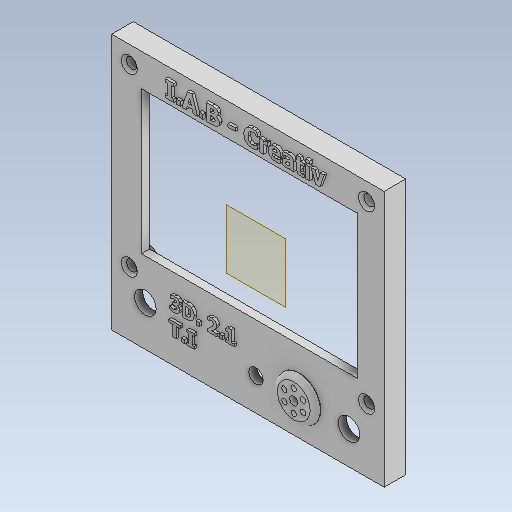
# Autodesk Inventor part: 10-06-005 carcasa Fata
Saved by Autodesk Inventor 2020 (Build 240168000, 168)
## iProperties
Created: 2019-11-09
Part Number: 10-06-005 carcasa Fata
Material: Generic
Document SubType Name: Modeling
Designer: iuliu
Density: 1 g/cm^3
Appearance: Default
Mass: 21.9353 g
Surface Area: 173.982 cm^2
Volume: 21.9353 cm^3
Description: Carcasa fata Display
Author: iuliu
Subject: 038
Autodesk Inventor part; units mm, degrees
ref_plane "YZ Plane" through (0, 0, 0) normal (1, 0, 0) x (0, 1, 0)
ref_plane "XZ Plane" through (0, 0, 0) normal (0, 1, 0) x (-1, 0, 0)
ref_plane "XY Plane" through (0, 0, 0) normal (0, 0, 1) x (1, 0, 0)
sketch "Sketch1" plane through (0, 0, 0) normal (0, 0, 1) x (1, 0, 0)
  line L0 (-50.5, 47.5) -> (50.5, 47.5)
  line L1 (50.5, 47.5) -> (50.5, -47.5)
  line L2 (50.5, -47.5) -> (-50.5, -47.5)
  line L3 (-50.5, -47.5) -> (-50.5, 47.5)
  point P0 (0, 0)
  point P1 (0, 47.5)
  point P2 (-50.5, 0)
  dimension "d0" = 95
  dimension "d1" = 101
  constraints: 8 end point, 2 midpoint, 2 parallel, 1 horizontal, 1 horizontal alignment, 1 perpendicular, 1 vertical alignment
  measures "d0" distance of L2.end L0.start
  measures "d1" distance of L0.start L0.end
extrude "Extrusion1" add sketch "Sketch1" along normal blind 8
ref_plane "Work Plane1" through (0, 0, 5) normal (0, 0, 1) x (1, 0, 0)
sketch "Sketch4" plane through (0, 0, 5) normal (0, 0, 1) x (1, 0, 0)
  circle A0 centre (-44, -24) radius 1.5 projected
  circle A1 centre (44, -24) radius 1.5 projected
  circle A2 centre (44, 41) radius 1.5 projected
  circle A3 centre (-44, 41) radius 1.5 projected
  circle A4 centre (-44, -24) radius 5
  circle A5 centre (44, -24) radius 5
  circle A6 centre (-44, 41) radius 5
  circle A7 centre (44, 41) radius 5
  point P0 (0, 0)
  dimension "d11" = 10
  dimension "d12" = 10
  dimension "d13" = 10
  dimension "d14" = 10
  constraints: 4 centre point, 4 coincident
  measures "d11" diameter of A4
  measures "d12" diameter of A5
  measures "d13" diameter of A6
  measures "d14" diameter of A7
hole "Hole1" at (-44, 41, 5) at (-44, -24, 5) at (44, 41, 5) at (44, -24, 5) direction (0, 0, -1) diameter 4 end through all both
sketch "Sketch5" plane through (0, 0, 0) normal (0, 0, -1) x (-1, 0, 0)
  line L0 (-3.5, 27) -> (-25.5, 27) projected
  line L1 (-25.5, 27) -> (-25.5, 38) projected
  line L2 (-25.5, 38) -> (-3.5, 38) projected
  line L3 (-3.5, 38) -> (-3.5, 27) projected
  line L4 (26.5, 27) -> (4.5, 27) projected
  line L5 (4.5, 27) -> (4.5, 38) projected
  line L6 (4.5, 38) -> (26.5, 38) projected
  line L7 (26.5, 38) -> (26.5, 27) projected
  line L8 (-50.5, -47.5) -> (-50.5, 47.5) projected
  line L9 (50.5, -47.5) -> (-50.5, -47.5) projected
  line L10 (50.5, 47.5) -> (50.5, -47.5) projected
  line L11 (-50.5, 47.5) -> (50.5, 47.5) projected
  line L12 (47.5, 44.5) -> (47.5, -44.5)
  line L13 (47.5, -44.5) -> (-47.5, -44.5)
  line L14 (-47.5, -44.5) -> (-47.5, 44.5)
  line L15 (-47.5, 44.5) -> (47.5, 44.5)
  circle A0 centre (0, -1.5) radius 2 projected
  circle A1 centre (0, -37.5) radius 2 projected
  point P0 (0, 0)
  dimension "d25" = 3
  constraints: 8 end point, 3 other
  measures "d25" distance between parallel lines of L11 L15
extrude "Extrusion5" cut sketch "Sketch5" against normal blind 5 contours L0 L1 L2 L3 | L4 L5 L6 L7 | L12 L13 L14 L15 | A0 | A1
sketch "Sketch6" plane through (0, 0, 5) normal (0, 0, -1) x (-1, 0, 0)
  circle A0 centre (-19, -34.5) radius 6 projected
  circle A1 centre (-3, -35.5) radius 1.65 projected
  circle A2 centre (38, -32.5) radius 3 projected
  line L0 (38.5, -16.5) -> (-39.5, -16.5) projected
  line L1 (-39.5, -16.5) -> (-39.5, 34.5) projected
  line L2 (38.5, 34.5) -> (38.5, -16.5) projected
  line L3 (-39.5, 34.5) -> (38.5, 34.5) projected
  circle A3 centre (-19, -34.5) radius 7
  circle A4 centre (-3, -35.5) radius 2.65
  circle A5 centre (38, -32.5) radius 4
  line L4 (39.5, 35.5) -> (39.5, -17.5)
  line L5 (39.5, -17.5) -> (-40.5, -17.5)
  line L6 (-40.5, -17.5) -> (-40.5, 35.5)
  line L7 (-40.5, 35.5) -> (39.5, 35.5)
  circle A6 centre (-37.5, -35.25) radius 3 projected
  circle A7 centre (-37.5, -35.25) radius 4
  point P0 (0, 0)
  dimension "d29" = 1
  dimension "d30" = 1
  dimension "d31" = 1
  dimension "d35" = 1
  dimension "d36" = 1
  constraints: 8 end point, 4 centre point, 3 other
  measures "d29" radial gap between concentric circles of A1 A4
  measures "d30" radial gap between concentric circles of A2 A5
  measures "d31" distance between parallel lines of L3 L7
  measures "d35" radial gap between concentric circles of A0 A3
  measures "d36" radial gap between concentric circles of A6 A7
extrude "Extrusion6" cut sketch "Sketch6" against normal through all contours A0 | A1 | A2 | L0 L1 L3 L2 | A3 | A4 | A5 | L4 L5 L6 L7 | A6 | A7
sketch "Sketch7" plane through (0, 0, 8) normal (0, 0, 1) x (1, 0, 0)
  circle A0 centre (19, -34.5) radius 7 projected
  circle A1 centre (19, -34.5) radius 8
  point P0 (0, 0)
  dimension "d71" = 14
  dimension "d72" = 16
  constraints: 1 centre point, 1 coincident
  measures "d71" diameter of A0
  measures "d72" diameter of A1
extrude "Extrusion7" add sketch "Sketch7" along normal blind 2 contours A0 | A1
sketch "Sketch8" plane through (19, -34.5, 10) normal (0, 0, 1) x (1, 0, 0)
  point P0 (-19, 34.5)
  point P1 (0, 0)
hole "Hole2" at (19, -34.5, 10) direction (0, 0, -1) diameter 3 end through all
sketch "Sketch9" plane through (19, -34.5, 10) normal (0, 0, 1) x (1, 0, 0)
  circle A0 centre (0, 0) radius 1.5 projected
  point P0 (-19, 34.5)
  point P1 (0, 4)
  dimension "d46" = 4
  constraints: 1 vertical alignment
  measures "d46" distance of A0.centre point (0, 4)
hole "Hole3" at (19, -30.5, 10) direction (0, 0, -1) diameter 2 end through all
pattern_circular "Circular Pattern1" count 6 over 360 about axis through (19, -34.5, 5) along (0, 0, 1) of "Hole3"
fillet "Fillet2" radius 1.9 1 edges at (11, -34.5, 10)
sketch "Sketch10" plane through (0, 0, 8) normal (0, 0, 1) x (1, 0, 0)
  circle A0 centre (-44, 41) radius 2 projected
  circle A1 centre (44, 41) radius 2 projected
  circle A2 centre (44, -24) radius 2 projected
  circle A3 centre (-44, -24) radius 2 projected
  point P0 (0, 0)
hole "Hole4" at (-44, 41, 8) at (44, 41, 8) at (44, -24, 8) at (-44, -24, 8) direction (0, 0, -1) diameter 4 end through all countersink diameter 6 countersink angle 90
sketch "Sketch11" plane through (0, 0, 8) normal (0, 0, 1) x (1, 0, 0)
  line L0 (-30.1228, 44.4062) -> (30.1228, 44.4062) construction
  line L1 (30.1228, 44.4062) -> (30.1228, 41.1581) construction
  line L2 (30.1228, 41.1581) -> (-30.1228, 41.1581) construction
  line L3 (-30.1228, 41.1581) -> (-30.1228, 44.4062) construction
  line L4 (-28.2931, -24.0933) -> (-3.3312, -24.0933) construction
  line L5 (-3.3312, -24.0933) -> (-3.3312, -28.0478) construction
  line L6 (-3.3312, -28.0478) -> (-28.2931, -28.0478) construction
  line L7 (-28.2931, -28.0478) -> (-28.2931, -24.0933) construction
  line L8 (50.5, 47.5) -> (-50.5, 47.5) projected
  line L9 (-26.4549, 38.0294) -> (-29.7372, 38.0294)
  line L10 (-29.7372, 38.0294) -> (-29.7372, 39.0922)
  line L11 (-29.7372, 39.0922) -> (-28.8623, 39.0922)
  line L12 (-28.8623, 39.0922) -> (-28.8623, 43.0666)
  line L13 (-28.8623, 43.0666) -> (-29.7372, 43.0666)
  line L14 (-29.7372, 43.0666) -> (-29.7372, 44.1294)
  line L15 (-29.7372, 44.1294) -> (-26.4549, 44.1294)
  line L16 (-26.4549, 44.1294) -> (-26.4549, 43.0666)
  line L17 (-26.4549, 43.0666) -> (-27.3298, 43.0666)
  line L18 (-27.3298, 43.0666) -> (-27.3298, 39.0922)
  line L19 (-27.3298, 39.0922) -> (-26.4549, 39.0922)
  line L20 (-26.4549, 39.0922) -> (-26.4549, 38.0294)
  line L21 (-24.0376, 38.0294) -> (-25.486, 38.0294)
  line L22 (-25.486, 38.0294) -> (-25.486, 39.6409)
  line L23 (-25.486, 39.6409) -> (-24.0376, 39.6409)
  line L24 (-24.0376, 39.6409) -> (-24.0376, 38.0294)
  line L25 (-23.4741, 38.0294) -> (-21.4127, 44.1294)
  line L26 (-21.4127, 44.1294) -> (-19.7419, 44.1294)
  line L27 (-19.7419, 44.1294) -> (-17.6806, 38.0294)
  line L28 (-17.6806, 38.0294) -> (-19.2575, 38.0294)
  line L29 (-19.2575, 38.0294) -> (-19.6381, 39.2751)
  line L30 (-19.6381, 39.2751) -> (-21.5561, 39.2751)
  line L31 (-21.5561, 39.2751) -> (-21.9417, 38.0294)
  line L32 (-21.9417, 38.0294) -> (-23.4741, 38.0294)
  line L33 (-19.9742, 40.3824) -> (-20.5971, 42.3992)
  line L34 (-20.5971, 42.3992) -> (-21.2249, 40.3824)
  line L35 (-21.2249, 40.3824) -> (-19.9742, 40.3824)
  line L36 (-15.6736, 38.0294) -> (-17.122, 38.0294)
  line L37 (-17.122, 38.0294) -> (-17.122, 39.6409)
  line L38 (-17.122, 39.6409) -> (-15.6736, 39.6409)
  line L39 (-15.6736, 39.6409) -> (-15.6736, 38.0294)
  spline S0 degree 2 poles (-9.5785, 39.8979) (-9.5785, 39.4432) (-9.9246, 38.756) (-10.2113, 38.5286) knots 0 0 0 1 2 2 2
  spline S1 degree 2 poles (-10.2113, 38.5286) (-10.5573, 38.2568) (-11.3779, 38.0294) (-12.0156, 38.0294) knots 0 0 0 1 2 2 2
  line L40 (-12.0156, 38.0294) -> (-14.4526, 38.0294)
  line L41 (-14.4526, 38.0294) -> (-14.4526, 44.1294)
  line L42 (-14.4526, 44.1294) -> (-12.3023, 44.1294)
  spline S2 degree 2 poles (-12.3023, 44.1294) (-11.63, 44.1294) (-10.9379, 44.0256) (-10.6364, 43.8624) knots 0 0 0 1 2 2 2
  spline S3 degree 2 poles (-10.6364, 43.8624) (-10.3052, 43.6894) (-9.9839, 43.0962) (-9.9839, 42.7107) knots 0 0 0 1 2 2 2
  spline S4 degree 2 poles (-9.9839, 42.7107) (-9.9839, 42.2658) (-10.4288, 41.5688) (-10.8242, 41.4056) knots 0 0 0 1 2 2 2
  line L43 (-10.8242, 41.4056) -> (-10.8242, 41.376)
  spline S5 degree 2 poles (-10.8242, 41.376) (-10.2558, 41.2573) (-9.5785, 40.5208) (-9.5785, 39.8979) knots 0 0 0 1 2 2 2
  spline S6 degree 2 poles (-11.1604, 39.9226) (-11.1604, 40.2094) (-11.3878, 40.5307) (-11.6152, 40.6147) knots 0 0 0 1 2 2 2
  spline S7 degree 2 poles (-11.6152, 40.6147) (-11.7536, 40.6691) (-12.243, 40.679) (-12.6483, 40.679) knots 0 0 0 1 2 2 2
  line L44 (-12.6483, 40.679) -> (-12.9301, 40.679)
  line L45 (-12.9301, 40.679) -> (-12.9301, 39.1416)
  line L46 (-12.9301, 39.1416) -> (-12.846, 39.1416)
  spline S8 degree 2 poles (-12.846, 39.1416) (-12.2529, 39.1416) (-11.7981, 39.1564) (-11.5608, 39.2603) knots 0 0 0 1 2 2 2
  spline S9 degree 2 poles (-11.5608, 39.2603) (-11.3532, 39.3542) (-11.1604, 39.7002) (-11.1604, 39.9226) knots 0 0 0 1 2 2 2
  spline S10 degree 2 poles (-11.541, 42.4091) (-11.541, 42.5574) (-11.6943, 42.8688) (-11.8524, 42.938) knots 0 0 0 1 2 2 2
  spline S11 degree 2 poles (-11.8524, 42.938) (-12.0007, 43.0073) (-12.416, 43.0171) (-12.8263, 43.0171) knots 0 0 0 1 2 2 2
  line L47 (-12.8263, 43.0171) -> (-12.9301, 43.0171)
  line L48 (-12.9301, 43.0171) -> (-12.9301, 41.722)
  line L49 (-12.9301, 41.722) -> (-12.7373, 41.722)
  spline S12 degree 2 poles (-12.7373, 41.722) (-12.3468, 41.722) (-12.0304, 41.7368) (-11.8623, 41.8159) knots 0 0 0 1 2 2 2
  spline S13 degree 2 poles (-11.8623, 41.8159) (-11.6794, 41.9049) (-11.541, 42.2064) (-11.541, 42.4091) knots 0 0 0 1 2 2 2
  line L50 (-3.7109, 40.155) -> (-6.4247, 40.155)
  line L51 (-6.4247, 40.155) -> (-6.4247, 41.2919)
  line L52 (-6.4247, 41.2919) -> (-3.7109, 41.2919)
  line L53 (-3.7109, 41.2919) -> (-3.7109, 40.155)
  spline S14 degree 2 poles (2.4633, 37.9107) (1.089, 37.9107) (-0.5225, 39.5717) (-0.5225, 41.0744) knots 0 0 0 1 2 2 2
  spline S15 degree 2 poles (-0.5225, 41.0744) (-0.5225, 42.5228) (1.094, 44.248) (2.4682, 44.248) knots 0 0 0 1 2 2 2
  spline S16 degree 2 poles (2.4682, 44.248) (2.8291, 44.248) (3.4124, 44.164) (3.6793, 44.0948) knots 0 0 0 1 2 2 2
  spline S17 degree 2 poles (3.6793, 44.0948) (3.8869, 44.0305) (4.3763, 43.8179) (4.5296, 43.7389) knots 0 0 0 1 2 2 2
  line L54 (4.5296, 43.7389) -> (4.5296, 42.2855)
  line L55 (4.5296, 42.2855) -> (4.3763, 42.2855)
  spline S18 degree 2 poles (4.3763, 42.2855) (4.2626, 42.3844) (3.9265, 42.6612) (3.7139, 42.7897) knots 0 0 0 1 2 2 2
  spline S19 degree 2 poles (3.7139, 42.7897) (3.5014, 42.9232) (2.9922, 43.1061) (2.7104, 43.1061) knots 0 0 0 1 2 2 2
  spline S20 degree 2 poles (2.7104, 43.1061) (2.3792, 43.1061) (1.8305, 42.8985) (1.5784, 42.6365) knots 0 0 0 1 2 2 2
  spline S21 degree 2 poles (1.5784, 42.6365) (1.351, 42.4042) (1.0594, 41.6083) (1.0594, 41.0695) knots 0 0 0 1 2 2 2
  spline S22 degree 2 poles (1.0594, 41.0695) (1.0594, 40.501) (1.3609, 39.7249) (1.6081, 39.4876) knots 0 0 0 1 2 2 2
  spline S23 degree 2 poles (1.6081, 39.4876) (1.8454, 39.2553) (2.4287, 39.0526) (2.7203, 39.0526) knots 0 0 0 1 2 2 2
  spline S24 degree 2 poles (2.7203, 39.0526) (3.0219, 39.0526) (3.5706, 39.2553) (3.7584, 39.3789) knots 0 0 0 1 2 2 2
  spline S25 degree 2 poles (3.7584, 39.3789) (3.966, 39.5025) (4.2775, 39.7645) (4.3912, 39.8683) knots 0 0 0 1 2 2 2
  line L56 (4.3912, 39.8683) -> (4.5296, 39.8683)
  line L57 (4.5296, 39.8683) -> (4.5296, 38.4347)
  spline S26 degree 2 poles (4.5296, 38.4347) (4.3615, 38.3556) (3.9215, 38.1579) (3.6843, 38.0887) knots 0 0 0 1 2 2 2
  spline S27 degree 2 poles (3.6843, 38.0887) (3.3976, 37.9997) (2.8983, 37.9107) (2.4633, 37.9107) knots 0 0 0 1 2 2 2
  line L58 (8.4397, 41.2722) -> (8.3211, 41.2722)
  spline S28 degree 2 poles (8.3211, 41.2722) (8.237, 41.3018) (7.9256, 41.3315) (7.7377, 41.3315) knots 0 0 0 1 2 2 2
  spline S29 degree 2 poles (7.7377, 41.3315) (7.5153, 41.3315) (7.016, 41.198) (6.7837, 41.109) knots 0 0 0 1 2 2 2
  line L59 (6.7837, 41.109) -> (6.7837, 38.0294)
  line L60 (6.7837, 38.0294) -> (5.3501, 38.0294)
  line L61 (5.3501, 38.0294) -> (5.3501, 42.6316)
  line L62 (5.3501, 42.6316) -> (6.7837, 42.6316)
  line L63 (6.7837, 42.6316) -> (6.7837, 41.9692)
  spline S30 degree 2 poles (6.7837, 41.9692) (6.8826, 42.0581) (7.2286, 42.335) (7.3719, 42.419) knots 0 0 0 1 2 2 2
  spline S31 degree 2 poles (7.3719, 42.419) (7.5301, 42.5129) (7.9454, 42.6464) (8.1283, 42.6464) knots 0 0 0 1 2 2 2
  spline S32 degree 2 poles (8.1283, 42.6464) (8.1975, 42.6464) (8.3705, 42.6365) (8.4397, 42.6316) knots 0 0 0 1 2 2 2
  line L64 (8.4397, 42.6316) -> (8.4397, 41.2722)
  spline S33 degree 2 poles (11.3463, 37.9058) (10.0413, 37.9058) (8.6523, 39.1515) (8.6523, 40.3033) knots 0 0 0 1 2 2 2
  spline S34 degree 2 poles (8.6523, 40.3033) (8.6523, 41.4303) (9.9474, 42.7749) (11.114, 42.7749) knots 0 0 0 1 2 2 2
  spline S35 degree 2 poles (11.114, 42.7749) (12.1669, 42.7749) (13.2347, 41.633) (13.2347, 40.5752) knots 0 0 0 1 2 2 2
  line L65 (13.2347, 40.5752) -> (13.2347, 40.0561)
  line L66 (13.2347, 40.0561) -> (10.0858, 40.0561)
  spline S36 degree 2 poles (10.0858, 40.0561) (10.1056, 39.7348) (10.3379, 39.3097) (10.5258, 39.1812) knots 0 0 0 1 2 2 2
  spline S37 degree 2 poles (10.5258, 39.1812) (10.7087, 39.0526) (11.203, 38.9439) (11.4946, 38.9439) knots 0 0 0 1 2 2 2
  spline S38 degree 2 poles (11.4946, 38.9439) (11.7418, 38.9439) (12.2262, 39.0526) (12.4289, 39.1466) knots 0 0 0 1 2 2 2
  spline S39 degree 2 poles (12.4289, 39.1466) (12.6069, 39.2207) (12.9035, 39.4036) (12.9974, 39.4728) knots 0 0 0 1 2 2 2
  line L67 (12.9974, 39.4728) -> (13.1506, 39.4728)
  line L68 (13.1506, 39.4728) -> (13.1506, 38.2864)
  spline S40 degree 2 poles (13.1506, 38.2864) (12.9727, 38.2172) (12.686, 38.0986) (12.4289, 38.0393) knots 0 0 0 1 2 2 2
  spline S41 degree 2 poles (12.4289, 38.0393) (12.1966, 37.975) (11.7023, 37.9058) (11.3463, 37.9058) knots 0 0 0 1 2 2 2
  spline S42 degree 2 poles (11.8209, 40.9212) (11.811, 41.376) (11.4106, 41.8555) (11.0003, 41.8555) knots 0 0 0 1 2 2 2
  spline S43 degree 2 poles (11.0003, 41.8555) (10.5801, 41.8555) (10.1056, 41.3513) (10.0809, 40.9212) knots 0 0 0 1 2 2 2
  line L69 (10.0809, 40.9212) -> (11.8209, 40.9212)
  spline S44 degree 2 poles (16.5071, 38.5188) (16.3588, 38.3952) (16.1265, 38.1974) (15.9288, 38.0986) knots 0 0 0 1 2 2 2
  spline S45 degree 2 poles (15.9288, 38.0986) (15.736, 38.0047) (15.3702, 37.9058) (15.0439, 37.9058) knots 0 0 0 1 2 2 2
  spline S46 degree 2 poles (15.0439, 37.9058) (14.4309, 37.9058) (13.6252, 38.7264) (13.6252, 39.3492) knots 0 0 0 1 2 2 2
  spline S47 degree 2 poles (13.6252, 39.3492) (13.6252, 39.8584) (14.0355, 40.4911) (14.4211, 40.674) knots 0 0 0 1 2 2 2
  spline S48 degree 2 poles (14.4211, 40.674) (14.8116, 40.8619) (15.8941, 41.0102) (16.517, 41.0497) knots 0 0 0 1 2 2 2
  line L70 (16.517, 41.0497) -> (16.517, 41.0744)
  spline S49 degree 2 poles (16.517, 41.0744) (16.517, 41.4551) (15.9535, 41.7467) (15.3899, 41.7467) knots 0 0 0 1 2 2 2
  spline S50 degree 2 poles (15.3899, 41.7467) (15.1378, 41.7467) (14.4557, 41.5638) (14.1343, 41.4205) knots 0 0 0 1 2 2 2
  line L71 (14.1343, 41.4205) -> (14.0108, 41.4205)
  line L72 (14.0108, 41.4205) -> (14.0108, 42.5327)
  spline S51 degree 2 poles (14.0108, 42.5327) (14.2233, 42.592) (15.1724, 42.7601) (15.6569, 42.7601) knots 0 0 0 1 2 2 2
  spline S52 degree 2 poles (15.6569, 42.7601) (16.8433, 42.7601) (17.9308, 41.9692) (17.9308, 41.1585) knots 0 0 0 1 2 2 2
  line L73 (17.9308, 41.1585) -> (17.9308, 38.0294)
  line L74 (17.9308, 38.0294) -> (16.5071, 38.0294)
  line L75 (16.5071, 38.0294) -> (16.5071, 38.5188)
  line L76 (16.5071, 39.2306) -> (16.5071, 40.1846)
  spline S53 degree 2 poles (16.5071, 40.1846) (16.1413, 40.15) (15.6915, 40.0957) (15.474, 40.0166) knots 0 0 0 1 2 2 2
  spline S54 degree 2 poles (15.474, 40.0166) (15.2812, 39.9523) (15.0736, 39.6854) (15.0736, 39.4679) knots 0 0 0 1 2 2 2
  spline S55 degree 2 poles (15.0736, 39.4679) (15.0736, 39.1466) (15.4245, 38.9043) (15.7656, 38.9043) knots 0 0 0 1 2 2 2
  spline S56 degree 2 poles (15.7656, 38.9043) (15.9535, 38.9043) (16.3489, 39.0773) (16.5071, 39.2306) knots 0 0 0 1 2 2 2
  spline S57 degree 2 poles (20.7534, 37.9404) (19.8784, 37.9404) (19.0776, 38.6621) (19.0776, 39.4827) knots 0 0 0 1 2 2 2
  line L77 (19.0776, 39.4827) -> (19.0776, 41.633)
  line L78 (19.0776, 41.633) -> (18.5289, 41.633)
  line L79 (18.5289, 41.633) -> (18.5289, 42.6316)
  line L80 (18.5289, 42.6316) -> (19.0776, 42.6316)
  line L81 (19.0776, 42.6316) -> (19.0776, 43.9465)
  line L82 (19.0776, 43.9465) -> (20.5112, 43.9465)
  line L83 (20.5112, 43.9465) -> (20.5112, 42.6316)
  line L84 (20.5112, 42.6316) -> (21.8953, 42.6316)
  line L85 (21.8953, 42.6316) -> (21.8953, 41.633)
  line L86 (21.8953, 41.633) -> (20.5112, 41.633)
  line L87 (20.5112, 41.633) -> (20.5112, 39.9968)
  spline S58 degree 2 poles (20.5112, 39.9968) (20.5112, 39.7546) (20.5211, 39.3937) (20.5804, 39.2504) knots 0 0 0 1 2 2 2
  spline S59 degree 2 poles (20.5804, 39.2504) (20.6397, 39.107) (20.9313, 38.9389) (21.2082, 38.9389) knots 0 0 0 1 2 2 2
  spline S60 degree 2 poles (21.2082, 38.9389) (21.3268, 38.9389) (21.6976, 39.0378) (21.7717, 39.0773) knots 0 0 0 1 2 2 2
  line L88 (21.7717, 39.0773) -> (21.8953, 39.0773)
  line L89 (21.8953, 39.0773) -> (21.8953, 38.0689)
  spline S61 degree 2 poles (21.8953, 38.0689) (21.6629, 38.0096) (21.139, 37.9404) (20.7534, 37.9404) knots 0 0 0 1 2 2 2
  line L90 (23.9121, 38.0294) -> (22.4786, 38.0294)
  line L91 (22.4786, 38.0294) -> (22.4786, 42.6316)
  line L92 (22.4786, 42.6316) -> (23.9121, 42.6316)
  line L93 (23.9121, 42.6316) -> (23.9121, 38.0294)
  line L94 (23.9566, 43.289) -> (22.439, 43.289)
  line L95 (22.439, 43.289) -> (22.439, 44.4062)
  line L96 (22.439, 44.4062) -> (23.9566, 44.4062)
  line L97 (23.9566, 44.4062) -> (23.9566, 43.289)
  line L98 (29.3151, 42.6316) -> (27.6641, 38.0294)
  line L99 (27.6641, 38.0294) -> (26.0971, 38.0294)
  line L100 (26.0971, 38.0294) -> (24.4608, 42.6316)
  line L101 (24.4608, 42.6316) -> (25.9685, 42.6316)
  line L102 (25.9685, 42.6316) -> (26.9078, 39.5914)
  line L103 (26.9078, 39.5914) -> (27.8371, 42.6316)
  line L104 (27.8371, 42.6316) -> (29.3151, 42.6316)
  spline S62 degree 2 poles (-24.2372, -27.6833) (-24.2372, -28.052) (-24.5087, -28.6557) (-24.7721, -28.8664) knots 0 0 0 1 2 2 2
  spline S63 degree 2 poles (-24.7721, -28.8664) (-25.0354, -29.0771) (-25.7526, -29.304) (-26.2672, -29.304) knots 0 0 0 1 2 2 2
  spline S64 degree 2 poles (-26.2672, -29.304) (-26.8507, -29.304) (-27.6854, -29.1095) (-27.9487, -28.988) knots 0 0 0 1 2 2 2
  line L105 (-27.9487, -28.988) -> (-27.9487, -27.9021)
  line L106 (-27.9487, -27.9021) -> (-27.8272, -27.9021)
  spline S65 degree 2 poles (-27.8272, -27.9021) (-27.5517, -28.0763) (-26.8102, -28.3356) (-26.5022, -28.3356) knots 0 0 0 1 2 2 2
  spline S66 degree 2 poles (-26.5022, -28.3356) (-26.3199, -28.3356) (-25.8944, -28.2708) (-25.7486, -28.1655) knots 0 0 0 1 2 2 2
  spline S67 degree 2 poles (-25.7486, -28.1655) (-25.6351, -28.0804) (-25.4974, -27.8332) (-25.4974, -27.6104) knots 0 0 0 1 2 2 2
  spline S68 degree 2 poles (-25.4974, -27.6104) (-25.4974, -27.3875) (-25.6918, -27.1484) (-25.8539, -27.0917) knots 0 0 0 1 2 2 2
  spline S69 degree 2 poles (-25.8539, -27.0917) (-26.016, -27.035) (-26.4658, -27.0228) (-26.64, -27.0228) knots 0 0 0 1 2 2 2
  line L107 (-26.64, -27.0228) -> (-26.8547, -27.0228)
  line L108 (-26.8547, -27.0228) -> (-26.8547, -26.1436)
  line L109 (-26.8547, -26.1436) -> (-26.6562, -26.1436)
  spline S70 degree 2 poles (-26.6562, -26.1436) (-26.4293, -26.1436) (-26.0444, -26.1031) (-25.9106, -26.0423) knots 0 0 0 1 2 2 2
  spline S71 degree 2 poles (-25.9106, -26.0423) (-25.7769, -25.9775) (-25.627, -25.7505) (-25.627, -25.5561) knots 0 0 0 1 2 2 2
  spline S72 degree 2 poles (-25.627, -25.5561) (-25.627, -25.4021) (-25.7688, -25.2116) (-25.8701, -25.159) knots 0 0 0 1 2 2 2
  spline S73 degree 2 poles (-25.8701, -25.159) (-25.9917, -25.0982) (-26.3158, -25.0577) (-26.4293, -25.0577) knots 0 0 0 1 2 2 2
  spline S74 degree 2 poles (-26.4293, -25.0577) (-26.6116, -25.0577) (-26.9965, -25.1428) (-27.1748, -25.2116) knots 0 0 0 1 2 2 2
  spline S75 degree 2 poles (-27.1748, -25.2116) (-27.3166, -25.2643) (-27.6246, -25.4345) (-27.6975, -25.4791) knots 0 0 0 1 2 2 2
  line L110 (-27.6975, -25.4791) -> (-27.8029, -25.4791)
  line L111 (-27.8029, -25.4791) -> (-27.8029, -24.4094)
  spline S76 degree 2 poles (-27.8029, -24.4094) (-27.5435, -24.3) (-26.6683, -24.0933) (-26.2105, -24.0933) knots 0 0 0 1 2 2 2
  spline S77 degree 2 poles (-26.2105, -24.0933) (-25.7648, -24.0933) (-25.1084, -24.2473) (-24.8774, -24.3972) knots 0 0 0 1 2 2 2
  spline S78 degree 2 poles (-24.8774, -24.3972) (-24.6222, -24.5552) (-24.3669, -25.0415) (-24.3669, -25.3454) knots 0 0 0 1 2 2 2
  spline S79 degree 2 poles (-24.3669, -25.3454) (-24.3669, -25.7749) (-24.8612, -26.4151) (-25.2664, -26.5082) knots 0 0 0 1 2 2 2
  line L112 (-25.2664, -26.5082) -> (-25.2664, -26.5569)
  spline S80 degree 2 poles (-25.2664, -26.5569) (-25.0881, -26.5812) (-24.7478, -26.7108) (-24.5857, -26.8567) knots 0 0 0 1 2 2 2
  spline S81 degree 2 poles (-24.5857, -26.8567) (-24.4358, -26.9864) (-24.2372, -27.3997) (-24.2372, -27.6833) knots 0 0 0 1 2 2 2
  spline S82 degree 2 poles (-18.9333, -26.7027) (-18.9333, -27.4037) (-19.5452, -28.5058) (-20.0111, -28.8016) knots 0 0 0 1 2 2 2
  spline S83 degree 2 poles (-20.0111, -28.8016) (-20.4001, -29.0528) (-21.3158, -29.1987) (-21.8304, -29.1987) knots 0 0 0 1 2 2 2
  line L113 (-21.8304, -29.1987) -> (-23.3944, -29.1987)
  line L114 (-23.3944, -29.1987) -> (-23.3944, -24.1987)
  line L115 (-23.3944, -24.1987) -> (-21.8466, -24.1987)
  spline S84 degree 2 poles (-21.8466, -24.1987) (-21.3199, -24.1987) (-20.4001, -24.3324) (-19.9949, -24.5917) knots 0 0 0 1 2 2 2
  spline S85 degree 2 poles (-19.9949, -24.5917) (-19.5047, -24.9078) (-18.9333, -25.9775) (-18.9333, -26.7027) knots 0 0 0 1 2 2 2
  spline S86 degree 2 poles (-20.2218, -26.6946) (-20.2218, -26.2003) (-20.5622, -25.4953) (-20.9106, -25.2967) knots 0 0 0 1 2 2 2
  spline S87 degree 2 poles (-20.9106, -25.2967) (-21.1659, -25.159) (-21.7251, -25.1306) (-22.1141, -25.1306) knots 0 0 0 1 2 2 2
  line L116 (-22.1141, -25.1306) -> (-22.1384, -25.1306)
  line L117 (-22.1384, -25.1306) -> (-22.1384, -28.2627)
  line L118 (-22.1384, -28.2627) -> (-22.1141, -28.2627)
  spline S88 degree 2 poles (-22.1141, -28.2627) (-21.6927, -28.2627) (-21.1132, -28.2343) (-20.8499, -28.0682) knots 0 0 0 1 2 2 2
  spline S89 degree 2 poles (-20.8499, -28.0682) (-20.5419, -27.8737) (-20.2218, -27.189) (-20.2218, -26.6946) knots 0 0 0 1 2 2 2
  line L119 (-17.0411, -29.1987) -> (-18.2283, -29.1987)
  line L120 (-18.2283, -29.1987) -> (-18.2283, -27.8778)
  line L121 (-18.2283, -27.8778) -> (-17.0411, -27.8778)
  line L122 (-17.0411, -27.8778) -> (-17.0411, -29.1987)
  line L123 (-10.3636, -29.1987) -> (-14.0387, -29.1987)
  line L124 (-14.0387, -29.1987) -> (-14.0387, -28.3843)
  spline S90 degree 2 poles (-14.0387, -28.3843) (-13.5727, -28.0115) (-12.8272, -27.3551) (-12.5476, -27.0593) knots 0 0 0 1 2 2 2
  spline S91 degree 2 poles (-12.5476, -27.0593) (-12.1789, -26.6744) (-11.8507, -26.0869) (-11.8507, -25.7789) knots 0 0 0 1 2 2 2
  spline S92 degree 2 poles (-11.8507, -25.7789) (-11.8507, -25.4304) (-12.268, -25.0577) (-12.6408, -25.0577) knots 0 0 0 1 2 2 2
  spline S93 degree 2 poles (-12.6408, -25.0577) (-12.8312, -25.0577) (-13.1716, -25.1509) (-13.3458, -25.2238) knots 0 0 0 1 2 2 2
  spline S94 degree 2 poles (-13.3458, -25.2238) (-13.516, -25.3008) (-13.7591, -25.4629) (-13.8199, -25.5034) knots 0 0 0 1 2 2 2
  line L125 (-13.8199, -25.5034) -> (-13.9171, -25.5034)
  line L126 (-13.9171, -25.5034) -> (-13.9171, -24.4134)
  spline S95 degree 2 poles (-13.9171, -24.4134) (-13.7064, -24.3121) (-12.8069, -24.1014) (-12.3896, -24.1014) knots 0 0 0 1 2 2 2
  spline S96 degree 2 poles (-12.3896, -24.1014) (-11.4982, -24.1014) (-10.5824, -24.8956) (-10.5824, -25.6128) knots 0 0 0 1 2 2 2
  spline S97 degree 2 poles (-10.5824, -25.6128) (-10.5824, -26.0544) (-10.9998, -26.9053) (-11.482, -27.3916) knots 0 0 0 1 2 2 2
  spline S98 degree 2 poles (-11.482, -27.3916) (-11.7859, -27.6914) (-12.3572, -28.1574) (-12.4828, -28.2546) knots 0 0 0 1 2 2 2
  line L127 (-12.4828, -28.2546) -> (-10.3636, -28.2546)
  line L128 (-10.3636, -28.2546) -> (-10.3636, -29.1987)
  line L129 (-8.4998, -29.1987) -> (-9.687, -29.1987)
  line L130 (-9.687, -29.1987) -> (-9.687, -27.8778)
  line L131 (-9.687, -27.8778) -> (-8.4998, -27.8778)
  line L132 (-8.4998, -27.8778) -> (-8.4998, -29.1987)
  line L133 (-4.0589, -29.1987) -> (-7.3612, -29.1987)
  line L134 (-7.3612, -29.1987) -> (-7.3612, -28.3275)
  line L135 (-7.3612, -28.3275) -> (-6.3077, -28.3275)
  line L136 (-6.3077, -28.3275) -> (-6.3077, -25.6817)
  line L137 (-6.3077, -25.6817) -> (-7.3612, -25.6817)
  line L138 (-7.3612, -25.6817) -> (-7.3612, -24.8672)
  spline S99 degree 2 poles (-7.3612, -24.8672) (-7.1303, -24.8672) (-6.6724, -24.8065) (-6.5346, -24.7416) knots 0 0 0 1 2 2 2
  spline S100 degree 2 poles (-6.5346, -24.7416) (-6.3766, -24.6606) (-6.1983, -24.3891) (-6.1821, -24.1865) knots 0 0 0 1 2 2 2
  line L139 (-6.1821, -24.1865) -> (-5.0881, -24.1865)
  line L140 (-5.0881, -24.1865) -> (-5.0881, -28.3275)
  line L141 (-5.0881, -28.3275) -> (-4.0589, -28.3275)
  line L142 (-4.0589, -28.3275) -> (-4.0589, -29.1987)
  line L143 (-26.8142, -37.4311) -> (-26.8142, -33.3832)
  line L144 (-26.8142, -33.3832) -> (-28.2931, -33.3832)
  line L145 (-28.2931, -33.3832) -> (-28.2931, -32.4311)
  line L146 (-28.2931, -32.4311) -> (-24.0792, -32.4311)
  line L147 (-24.0792, -32.4311) -> (-24.0792, -33.3832)
  line L148 (-24.0792, -33.3832) -> (-25.5581, -33.3832)
  line L149 (-25.5581, -33.3832) -> (-25.5581, -37.4311)
  line L150 (-25.5581, -37.4311) -> (-26.8142, -37.4311)
  line L151 (-22.4179, -37.4311) -> (-23.6051, -37.4311)
  line L152 (-23.6051, -37.4311) -> (-23.6051, -36.1101)
  line L153 (-23.6051, -36.1101) -> (-22.4179, -36.1101)
  line L154 (-22.4179, -36.1101) -> (-22.4179, -37.4311)
  line L155 (-18.9293, -37.4311) -> (-21.6197, -37.4311)
  line L156 (-21.6197, -37.4311) -> (-21.6197, -36.5599)
  line L157 (-21.6197, -36.5599) -> (-20.9025, -36.5599)
  line L158 (-20.9025, -36.5599) -> (-20.9025, -33.3022)
  line L159 (-20.9025, -33.3022) -> (-21.6197, -33.3022)
  line L160 (-21.6197, -33.3022) -> (-21.6197, -32.4311)
  line L161 (-21.6197, -32.4311) -> (-18.9293, -32.4311)
  line L162 (-18.9293, -32.4311) -> (-18.9293, -33.3022)
  line L163 (-18.9293, -33.3022) -> (-19.6465, -33.3022)
  line L164 (-19.6465, -33.3022) -> (-19.6465, -36.5599)
  line L165 (-19.6465, -36.5599) -> (-18.9293, -36.5599)
  line L166 (-18.9293, -36.5599) -> (-18.9293, -37.4311)
  point P0 (0, 0)
  point P1 (0, 44.4062)
  point P2 (0, 47.5)
  constraints: 2 midpoint, 1 vertical alignment, 4 other
extrude "Extrusion8" add sketch "Sketch11" along normal blind 1
sketch "Sketch12" plane through (0, 0, 5) normal (0, 0, -1) x (-1, 0, 0)
  circle A0 centre (-44, 41) radius 4
  circle A1 centre (44, 41) radius 4
  circle A2 centre (44, -24) radius 4
  circle A3 centre (-44, -24) radius 4
  circle A4 centre (-44, 41) radius 2 projected
  circle A5 centre (44, 41) radius 2 projected
  circle A6 centre (44, -24) radius 2 projected
  circle A7 centre (-44, -24) radius 2 projected
  point P0 (0, 0)
  dimension "d67" = 8
  constraints: 4 centre point, 4 concentric, 3 equal radius
  measures "d67" diameter of A0
extrude "Extrusion9" add sketch "Sketch12" along normal blind 4
fillet "Fillet3" radius 2 8 edges at (47.5, 39.0635, 3) (42.0635, 44.5, 3) (-42.0635, 44.5, 3) (-47.5, 39.0635, 3) (-47.5, -22.0635, 3) (-47.5, -25.9365, 3) (47.5, -25.9365, 3) (47.5, -22.0635, 3)
body "Solid1"
